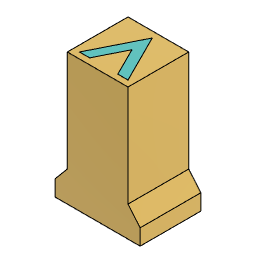
Key_Up_Down (Autodesk Fusion 360 design; units mm, degrees)
Autodesk Fusion 360 part; units mm, degrees
sketch "Skizze1" plane through (0, 0, 0) normal (0, 0, 1) x (1, 0, 0) in component "Key_Up_Down"
  line L0 (5, -5) -> (-5, -5)
  line L1 (-5, -5) -> (-5, 5)
  line L2 (-5, 5) -> (5, 5)
  line L3 (5, 5) -> (5, -5)
  line L4 (5, -5) -> (-5, 5) construction
  line L5 (-5, -5) -> (5, 5) construction
  dimension "d1" = 10
  dimension "d2" = 10
  constraint horizontal L0
  constraint perpendicular L0 L1
  constraint parallel L0 L2
  constraint parallel L1 L3
  constraint coincident L4 origin
  constraint coincident L5 origin
  measures "d1" distance of L1.end L2.end
  measures "d2" distance of L0.end L1.end
extrude "Extrusion1" add sketch "Skizze1" along normal blind 21.7 makes body 1 in component "Key_Up_Down"
sketch "Skizze2" plane through (0, 0, 21.7) normal (0, 0, 1) x (-1, 0, 0) in component "Key_Up_Down"
  line L0 (-5, -5) -> (5, -5)
  line L1 (5, -5) -> (5, 5)
  line L2 (5, 5) -> (-5, 5)
  line L3 (-5, 5) -> (-5, -5)
  line L4 (0, -4) -> (4, 4.0007)
  line L5 (4, 4.0007) -> (2.323, 4.0007)
  line L6 (2.323, 4.0007) -> (0, -0.6457)
  line L7 (0, -0.6457) -> (-2.3243, 4)
  line L8 (-2.3243, 4) -> (-4.0013, 4)
  line L9 (-4.0013, 4) -> (0, -4)
  dimension "d5" = 1
  dimension "d6" = 1
  dimension "d7" = 1
  dimension "d8" = 1.5
  constraint horizontal L5
  constraint parallel L4 L6
  constraint parallel L5 L8
  constraint equal L4 L9
  constraint equal L5 L8
  constraint vertical origin L6.end
  constraint vertical origin L4.start
  constraint equal L6 L7
  measures "d5" distance of L0 L4.start
  measures "d6" distance of L2 L8
  measures "d7" distance of L1 L4.end
  measures "d8" distance of L4 L6
extrude "Extrusion2" cut sketch "Skizze2" against normal blind 0.5 contours L4 L5 L6 L7 L8 L9 bodies 1 in component "Key_Up_Down"
extrude "Extrusion1'" add 1 faces at (1.3338, 0.2152, 21.2) along direction (0, 0, 1) up to surface (0.5 mm away) separate body on bodies 1 makes body 2 in component "Key_Up_Down_Icon"
sketch "Skizze3" plane through (0, -5, 0) normal (0, -1, 0) x (1, 0, 0) in component "Key_Up_Down"
  line L0 (-5, 0) -> (5, 0)
  line L1 (5, 0) -> (5, 21.7)
  line L2 (5, 21.7) -> (-5, 21.7)
  line L3 (-5, 21.7) -> (-5, 0)
  line L4 (5, 0) -> (7, 0)
  line L5 (7, 0) -> (7, 2.6165)
  line L6 (7, 2.6165) -> (5, 5)
  line L7 (0, 20) -> (0, 2.5)
  line L8 (-5, 0) -> (-7, 0)
  line L9 (-7, 2.6165) -> (-5, 5)
  line L10 (-7, 0) -> (-7, 2.6165)
  point P0 (-5, 0)
  dimension "d19" = 2
  dimension "d20" = 5
  dimension "d21" = 40
  constraint coincident L0.end L1.start
  constraint perpendicular L1 L4
  constraint perpendicular L4 L5
  constraint coincident L1 L6.end
  constraint symmetric L0.end L7 P0
  constraint symmetric L4.end L7 L8.end
  constraint symmetric L5.end L7 L9.start
  constraint symmetric L6.end L7 L9.end
  measures "d19" distance of L0.end L4.end
  measures "d20" distance of L0.end L6.end
  measures "d21" angle of L1 L6
extrude "Extrusion4" add sketch "Skizze3" against normal up to surface (10 mm away) contours L3 L8 L9 L10 | L1 L4 L5 L6 bodies 1 in component "Key_Up_Down"
component "Key_Up_Down" placed x (1, 0, 0) y (0, 1, 0) z (0, 0, 1) at (0, 0, 0)
component "Key_Up_Down_Icon" placed x (1, 0, 0) y (0, 1, 0) z (0, 0, 1) at (0, 0, 0)
equation "d6 = d5"
equation "d7 = d5"
